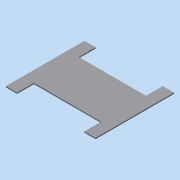
# Autodesk Inventor part: Platte
Saved by Autodesk Inventor 2014 SP2 (Build 180246200, 246)
## iProperties
Created: 2015-10-03
Part Number: Platte
Material: Generisch
Document SubType Name: Modeling
Designer: Home
Density: 1 g/cm^3
Appearance: Vorgabe
Author: Home
Autodesk Inventor part; units mm, degrees
ref_plane "YZ Plane" through (0, 0, 0) normal (1, 0, 0) x (0, 1, 0)
ref_plane "XZ Plane" through (0, 0, 0) normal (0, 1, 0) x (-1, 0, 0)
ref_plane "XY Plane" through (0, 0, 0) normal (0, 0, 1) x (1, 0, 0)
sketch "Skizze1" plane through (0, 0, 0) normal (0, 0, 1) x (1, 0, 0)
  line L0 (-150, 100) -> (150, 100)
  line L1 (200, 100) -> (200, -100)
  line L2 (150, -100) -> (-150, -100)
  line L3 (-200, -100) -> (-200, 100)
  line L4 (-305.5062, 0) -> (363.7655, 0) construction
  line L5 (0, 250.7333) -> (0, -254.4177) construction
  line L6 (-200, 100) -> (-150, 100)
  line L7 (-150, 100) -> (-150, 175)
  line L8 (-150, 175) -> (-200, 175)
  line L9 (-200, 175) -> (-200, 100)
  line L10 (150, 100) -> (150, 175)
  line L11 (150, 175) -> (200, 175)
  line L12 (200, 175) -> (200, 100)
  line L13 (-150, -100) -> (-150, -175)
  line L14 (-150, -175) -> (-200, -175)
  line L15 (-200, -175) -> (-200, -100)
  line L16 (150, -175) -> (200, -175)
  line L17 (150, -100) -> (150, -175)
  line L18 (200, -175) -> (200, -100)
  point P0 (0, 0)
  dimension "d0" = 400
  dimension "d1" = 200
  dimension "d2" = 50
  dimension "d3" = 75
  constraints: 38 end point, 9 symmetric about line, 4 parallel, 4 perpendicular, 2 horizontal, 2 point on line, 2 other
  measures "d0" distance of L3.end L1.start
  measures "d1" distance of L3.start L3.end
  measures "d2" distance of L7.end L8.end
  measures "d3" distance of L8.end L3.end
extrude "Extrusion1" add sketch "Skizze1" along normal blind 5
